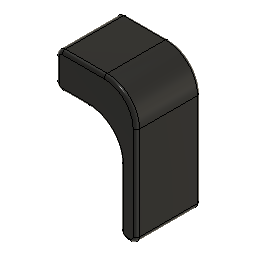
Arm Strap Support2 (Autodesk Fusion 360 design; units mm, degrees)
Autodesk Fusion 360 part; units mm, degrees
sketch "Sketch1" plane through (0, 57.15, 0) normal (0, 1, 0) x (-1, 0, 0)
  line L0 (-4.0409, -6.0198) -> (-4.0409, -7.62)
  line L1 (-4.0409, -7.62) -> (2.9359, -7.62)
  line L2 (2.9359, -7.62) -> (2.9359, -6.0198)
  line L3 (2.9359, -6.0198) -> (-4.0409, -6.0198)
  line L4 (-19.0526, 3.8099) -> (-19.0526, -5.08)
  line L5 (-21.5926, -7.62) -> (-31.7526, -7.62)
  line L6 (-44.4526, -7.62) -> (-44.4526, 6.3499)
  line L7 (-44.4526, 6.3499) -> (-21.5926, 6.3499)
  line L8 (-44.4526, -20.32) -> (-44.4526, -43.18)
  line L9 (-46.9926, -45.72) -> (-48.2626, -45.72)
  line L10 (-50.8026, -43.18) -> (-50.8026, -6.3501)
  line L11 (-38.1026, 6.3499) -> (-44.4526, 6.3499)
  arc A0 (-19.0526, 3.8099) -> (-21.5926, 6.3499) centre (-21.5926, 3.8099) ccw
  arc A1 (-21.5926, -7.62) -> (-19.0526, -5.08) centre (-21.5926, -5.08) ccw
  arc A2 (-46.9926, -45.72) -> (-44.4526, -43.18) centre (-46.9926, -43.18) ccw
  arc A3 (-50.8026, -43.18) -> (-48.2626, -45.72) centre (-48.2626, -43.18) ccw
  arc A4 (-31.7526, -7.62) -> (-44.4526, -20.32) centre (-31.7526, -20.32) ccw
  arc A5 (-38.1026, 6.3499) -> (-50.8026, -6.3501) centre (-38.1026, -6.3501) ccw
  point P0 (-19.0526, -7.62)
  point P1 (-44.4526, -45.72)
  point P2 (-50.8026, -45.72)
  dimension "d1" = 25.4
  dimension "d2" = 38.1
  dimension "d3" = 6.35
  dimension "d4" = 2.54
  dimension "d5" = 2.54
  dimension "d6" = 12.7
  constraint perpendicular L1 L4
  constraint perpendicular L4 L5
  constraint perpendicular L5 L6
  constraint perpendicular L4 L7
  constraint perpendicular L5 L8
  constraint perpendicular L8 L9
  constraint perpendicular L9 L10
  constraint perpendicular L6 L11
  constraint tangent L4 A0
  constraint tangent L7 A0
  constraint coincident P0 L4
  constraint coincident P0 L5
  constraint tangent L4 A1
  constraint tangent L5 A1
  constraint equal A0 A1
  constraint coincident P1 L8
  constraint coincident P1 L9
  constraint tangent L8 A2
  constraint tangent L9 A2
  constraint coincident P2 L9
  constraint coincident P2 L10
  constraint tangent L9 A3
  constraint tangent L10 A3
  constraint equal A2 A3
  constraint coincident L6.start L5
  constraint coincident L6.start L8
  constraint tangent L5 A4
  constraint tangent L8 A4
  constraint tangent L10 A5
  constraint tangent L11 A5
  constraint equal A4 A5
  measures "d1" distance of P0 L6.start
  measures "d2" distance of L6.start P1
  measures "d3" distance of P1 P2
  measures "d4" radius of A0
  measures "d5" radius of A2
  measures "d6" radius of A4
extrude "Extrude1" add sketch "Sketch1" against normal blind 25.4 contours L4 L5 L7 L8 L9 L10 A0 A1 A2 A3 A4 A5
fillet "Fillet1" radius 1.27 12 edges at (19.0526, 31.75, -0.6351) (19.7966, 31.75, -6.8761) (26.6726, 31.75, -7.62) (40.7329, 31.75, -11.3397) (44.4526, 31.75, -31.75) (45.1966, 31.75, -44.9761) (47.6276, 31.75, -45.72) (50.0587, 31.75, -44.9761) (50.8026, 31.75, -24.7651) (47.0829, 31.75, 2.6301) (29.8476, 31.75, 6.3499) (19.7966, 31.75, 5.6059) 1 faces at (30.4826, 57.15, 1.6932)
hole "Hole4" at (19.0526, 50.8, 0) direction (1, 0, 0) diameter 3.429 depth 12.7 tip angle 180
thread "Thread4" "ANSI Unified Screw Threads 0.164(#8) 8-32 UNC 8-32 UNC 2B" major diameter 4.1656 minor diameter 3.4163 pitch 0.7937 angle 60 modelled right hand crest width 0.2341 on face at (23.2859, 50.9707, 1.706) crest through (19.251, 49.0918, 0)
hole "Hole5" at (19.0526, 38.1, 0) direction (1, 0, 0) diameter 3.429 depth 12.7 tip angle 180
thread "Thread5" "ANSI Unified Screw Threads 0.164(#8) 8-32 UNC 8-32 UNC 2B" major diameter 4.1656 minor diameter 3.4163 pitch 0.7937 angle 60 modelled right hand crest width 0.2341 on face at (23.2859, 38.2707, 1.706) crest through (19.251, 36.3918, 0)
sketch "Sketch2" plane through (19.0526, 0, 0) normal (-1, 0, 0) x (0, -1, 0)
  spline S0 degree 3 poles (-39.1037, -1.825) (-39.3209, -1.674) (-39.5071, -1.4829) (-39.7881, -1.048) (-39.8836, -0.8108) (-39.9744, -0.3235) (-39.9728, -0.0789) (-39.8889, 0.3235) (-39.8315, 0.4832) (-39.6758, 0.7763) (-39.5795, 0.909) (-39.4657, 1.0259) knots 0 0 0 0 0.079347 0.079347 0.155456 0.155456 0.228326 0.228326 0.279114 0.279114 0.328226 0.328226 0.328226 0.328226
  arc A0 (-36.7343, 1.0259) -> (-39.4657, 1.0259) centre (-38.1, 0) ccw
  spline S1 degree 3 poles (-36.7343, 1.0259) (-36.5767, 0.864) (-36.4531, 0.6723) (-36.2803, 0.2427) (-36.2366, 0.0074) (-36.2398, -0.4776) (-36.2908, -0.7228) (-36.4588, -1.1248) (-36.5557, -1.2864) (-36.7951, -1.5826) (-36.9376, -1.7147) (-37.0963, -1.825) knots 0 0 0 0 0.06777 0.06777 0.138771 0.138771 0.213001 0.213001 0.26909 0.26909 0.326867 0.326867 0.326867 0.326867
  arc A1 (-39.1037, -1.825) -> (-37.0963, -1.825) centre (-38.1, 0) ccw
  spline S2 degree 3 poles (-51.8037, -1.825) (-52.0209, -1.674) (-52.2071, -1.4829) (-52.4881, -1.048) (-52.5836, -0.8108) (-52.6744, -0.3235) (-52.6728, -0.0789) (-52.5889, 0.3235) (-52.5315, 0.4832) (-52.3758, 0.7763) (-52.2795, 0.909) (-52.1657, 1.0259) knots 0 0 0 0 0.079347 0.079347 0.155456 0.155456 0.228326 0.228326 0.279114 0.279114 0.328226 0.328226 0.328226 0.328226
  arc A2 (-49.4343, 1.0259) -> (-52.1657, 1.0259) centre (-50.8, 0) ccw
  spline S3 degree 3 poles (-49.4343, 1.0259) (-49.2767, 0.864) (-49.1531, 0.6723) (-48.9803, 0.2427) (-48.9366, 0.0074) (-48.9398, -0.4776) (-48.9908, -0.7228) (-49.1588, -1.1248) (-49.2557, -1.2864) (-49.4951, -1.5826) (-49.6376, -1.7147) (-49.7963, -1.825) knots 0 0 0 0 0.06777 0.06777 0.138771 0.138771 0.213001 0.213001 0.26909 0.26909 0.326867 0.326867 0.326867 0.326867
  arc A3 (-51.8037, -1.825) -> (-49.7963, -1.825) centre (-50.8, 0) ccw
  line L0 (-55.88, 3.8099) -> (-55.88, -5.08)
  line L1 (-55.88, -5.08) -> (-33.02, -5.08)
  line L2 (-33.02, -5.08) -> (-33.02, 3.8099)
  line L3 (-33.02, 3.8099) -> (-55.88, 3.8099)
  line L4 (-35.7886, 0) -> (-35.7886, 1.8034)
  line L5 (-36.2966, 2.3114) -> (-39.9034, 2.3114)
  line L6 (-40.4114, 1.8034) -> (-40.4114, -1.8034)
  line L7 (-39.9034, -2.3114) -> (-36.2966, -2.3114)
  line L8 (-35.7886, -1.8034) -> (-35.7886, 0)
  arc A4 (-35.7886, 1.8034) -> (-36.2966, 2.3114) centre (-36.2966, 1.8034) ccw
  arc A5 (-36.2966, -2.3114) -> (-35.7886, -1.8034) centre (-36.2966, -1.8034) ccw
  arc A6 (-40.4114, -1.8034) -> (-39.9034, -2.3114) centre (-39.9034, -1.8034) ccw
  arc A7 (-39.9034, 2.3114) -> (-40.4114, 1.8034) centre (-39.9034, 1.8034) ccw
  line L9 (-40.3987, 1.8034) -> (-40.3987, -1.8034)
  arc A8 (-40.3987, -1.8034) -> (-39.9034, -2.2987) centre (-39.9034, -1.8034) ccw
  line L10 (-39.9034, -2.2987) -> (-36.2966, -2.2987)
  arc A9 (-36.2966, -2.2987) -> (-35.8013, -1.8034) centre (-36.2966, -1.8034) ccw
  line L11 (-35.8013, -1.8034) -> (-35.8013, 0)
  line L12 (-35.8013, 0) -> (-35.8013, 1.8034)
  arc A10 (-35.8013, 1.8034) -> (-36.2966, 2.2987) centre (-36.2966, 1.8034) ccw
  line L13 (-36.2966, 2.2987) -> (-39.9034, 2.2987)
  arc A11 (-39.9034, 2.2987) -> (-40.3987, 1.8034) centre (-39.9034, 1.8034) ccw
  line L14 (-40.1447, 1.8034) -> (-40.1447, -1.8034)
  arc A12 (-40.1447, -1.8034) -> (-39.9034, -2.0447) centre (-39.9034, -1.8034) ccw
  line L15 (-39.9034, -2.0447) -> (-36.2966, -2.0447)
  arc A13 (-36.2966, -2.0447) -> (-36.0553, -1.8034) centre (-36.2966, -1.8034) ccw
  line L16 (-36.0553, -1.8034) -> (-36.0553, 0)
  line L17 (-36.0553, 0) -> (-36.0553, 1.8034)
  arc A14 (-36.0553, 1.8034) -> (-36.2966, 2.0447) centre (-36.2966, 1.8034) ccw
  line L18 (-36.2966, 2.0447) -> (-39.9034, 2.0447)
  arc A15 (-39.9034, 2.0447) -> (-40.1447, 1.8034) centre (-39.9034, 1.8034) ccw
  line L19 (-48.9966, 2.2987) -> (-52.6034, 2.2987)
  arc A16 (-52.6034, 2.2987) -> (-53.0987, 1.8034) centre (-52.6034, 1.8034) ccw
  line L20 (-53.0987, 1.8034) -> (-53.0987, -1.8034)
  arc A17 (-53.0987, -1.8034) -> (-52.6034, -2.2987) centre (-52.6034, -1.8034) ccw
  line L21 (-52.6034, -2.2987) -> (-48.9966, -2.2987)
  arc A18 (-48.9966, -2.2987) -> (-48.5013, -1.8034) centre (-48.9966, -1.8034) ccw
  line L22 (-48.5013, -1.8034) -> (-48.5013, 0)
  line L23 (-48.5013, 0) -> (-48.5013, 1.8034)
  arc A19 (-48.5013, 1.8034) -> (-48.9966, 2.2987) centre (-48.9966, 1.8034) ccw
  line L24 (-48.9966, 2.0447) -> (-52.6034, 2.0447)
  arc A20 (-48.7553, 1.8034) -> (-48.9966, 2.0447) centre (-48.9966, 1.8034) ccw
  line L25 (-48.7553, 0) -> (-48.7553, 1.8034)
  line L26 (-48.7553, -1.8034) -> (-48.7553, 0)
  arc A21 (-48.9966, -2.0447) -> (-48.7553, -1.8034) centre (-48.9966, -1.8034) ccw
  line L27 (-52.6034, -2.0447) -> (-48.9966, -2.0447)
  line L28 (-52.8447, 1.8034) -> (-52.8447, -1.8034)
  arc A22 (-52.8447, -1.8034) -> (-52.6034, -2.0447) centre (-52.6034, -1.8034) ccw
  arc A23 (-52.6034, 2.0447) -> (-52.8447, 1.8034) centre (-52.6034, 1.8034) ccw
  point P0 (-35.7886, 2.3114)
  point P1 (-40.4114, 2.3114)
  point P2 (-40.4114, -2.3114)
  dimension "d40" = 2.3114
  dimension "d41" = 2.3114
  dimension "d42" = 4.6228
  dimension "d43" = 4.6228
  dimension "d44" = 0.508
  dimension "d45" = -0.0127
  dimension "d46" = -0.254
  dimension "d49" = -12.7
  dimension "d50" = 0
  constraint perpendicular L4 L5
  constraint perpendicular L6 L7
  constraint coincident P0 L4
  constraint coincident P0 L5
  constraint tangent L4 A4
  constraint tangent L5 A4
  constraint tangent L7 A5
  constraint tangent L8 A5
  constraint equal A4 A5
  constraint coincident P2 L6
  constraint coincident P2 L7
  constraint tangent L6 A6
  constraint tangent L7 A6
  constraint equal A4 A6
  constraint coincident P1 L5
  constraint coincident P1 L6
  constraint tangent L5 A7
  constraint tangent L6 A7
  constraint equal A4 A7
  measures "d40" distance of A0.centre L4.start
  measures "d41" distance of L4.start P0
  measures "d42" distance of P0 P1
  measures "d43" distance of P1 P2
  measures "d44" radius of A4
equation "d42 = ( 0.091 * 2 ) * 1 in"
equation "d43 = ( 0.091 * 2 ) * 1 in"
named bodies: "ArmSupport2"
